Autodesk Inventor part; units mm, degrees
(part 3 of 3)
sketch "Эскиз8" plane through (0, 0, 0) normal (-1, 0, 0) x (0, 0, 1)
  circle A0 centre (-20, 29) radius 1.75 projected
  line L0 (-20, 32.1) -> (-17.3153, 30.55)
  line L1 (-17.3153, 30.55) -> (-17.3153, 27.45)
  line L2 (-17.3153, 27.45) -> (-20, 25.9)
  line L3 (-20, 25.9) -> (-22.6847, 27.45)
  line L4 (-22.6847, 27.45) -> (-22.6847, 30.55)
  line L5 (-22.6847, 30.55) -> (-20, 32.1)
  circle A1 centre (-10, 29) radius 1.75 projected
  line L6 (-10, 32.1) -> (-7.3153, 30.55)
  line L7 (-7.3153, 30.55) -> (-7.3153, 27.45)
  line L8 (-7.3153, 27.45) -> (-10, 25.9)
  line L9 (-10, 25.9) -> (-12.6847, 27.45)
  line L10 (-12.6847, 27.45) -> (-12.6847, 30.55)
  line L11 (-12.6847, 30.55) -> (-10, 32.1)
  circle A2 centre (10, 29) radius 1.75 projected
  line L12 (10, 32.1) -> (12.6847, 30.55)
  line L13 (12.6847, 30.55) -> (12.6847, 27.45)
  line L14 (12.6847, 27.45) -> (10, 25.9)
  line L15 (10, 25.9) -> (7.3153, 27.45)
  line L16 (7.3153, 27.45) -> (7.3153, 30.55)
  line L17 (7.3153, 30.55) -> (10, 32.1)
  circle A3 centre (20, 29) radius 1.75 projected
  line L18 (20, 32.1) -> (22.6847, 30.55)
  line L19 (22.6847, 30.55) -> (22.6847, 27.45)
  line L20 (22.6847, 27.45) -> (20, 25.9)
  line L21 (20, 25.9) -> (17.3153, 27.45)
  line L22 (17.3153, 27.45) -> (17.3153, 30.55)
  line L23 (17.3153, 30.55) -> (20, 32.1)
  point P0 (0, 0)
  dimension "d48" = 6.2
  dimension "d49" = 6.2
  dimension "d50" = 6.2
  dimension "d51" = 6.2
  constraints: 48 end point, 4 coincident, 52 other
  measures "d48" distance of L2.end L0.start
  measures "d49" distance of L8.end L6.start
  measures "d50" distance of L14.end L12.start
  measures "d51" distance of L20.end L18.start
extrude "Выдавливание8" cut sketch "Эскиз8" against normal blind 2.5
chamfer "Фаска1" distance 4 angle 45 2 edges at (10, -56.5, 36.5) (10, -56.5, -43.5)
equation "\"d13\" = d12"
equation "\"d14\" = d12"
equation "\"d15\" = d12"
equation "\"d6\" = d4"
equation "\"d7\" = d5"
equation "\"d8\" = d5"
equation "\"d9\" = d4"
equation "\"d10\" = d5"
equation "\"d11\" = d4"
equation "\"d38\" = d39"
equation "\"d40\" = d42"
equation "\"d41\" = d39"
equation "\"d43\" = d42"
equation "\"d44\" = d39"
equation "\"d45\" = d42"
equation "\"d49\" = d48"
equation "\"d50\" = d48"
equation "\"d51\" = d48"
